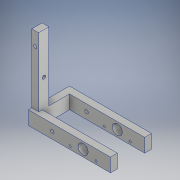
# Autodesk Inventor part: shooter
Saved by Autodesk Inventor 2019 (Build 230136000, 136)
## iProperties
Created: 2019-04-02
Part Number: shooter
Material: Aluminum 6061
Document SubType Name: Modeling
Designer: User
Density: 2.7 g/cm^3
Appearance: Aluminum - Flat
Mass: 367.89 g
Surface Area: 375.999 cm^2
Volume: 136.256 cm^3
Author: User
Autodesk Inventor part; units mm, degrees
ref_plane "YZ Plane" through (0, 0, 0) normal (1, 0, 0) x (0, 1, 0)
ref_plane "XZ Plane" through (0, 0, 0) normal (0, 1, 0) x (-1, 0, 0)
ref_plane "XY Plane" through (0, 0, 0) normal (0, 0, 1) x (1, 0, 0)
sketch "Sketch1" plane through (0, 0, 0) normal (1, 0, 0) x (0, 1, 0)
  line L0 (0, 0) -> (-152.4, 0)
  line L1 (-152.4, 0) -> (-152.4, -12.7)
  line L2 (-152.4, -12.7) -> (0, -12.7)
  line L3 (0, -12.7) -> (0, 0)
  line L4 (0, -12.7) -> (-12.7, -12.7)
  line L5 (-12.7, -12.7) -> (-12.7, -63.5)
  line L6 (-12.7, -63.5) -> (0, -63.5)
  line L7 (0, -63.5) -> (0, -12.7)
  line L8 (0, -63.5) -> (-152.4, -63.5)
  line L9 (-152.4, -63.5) -> (-152.4, -76.2)
  line L10 (-152.4, -76.2) -> (0, -76.2)
  line L11 (0, -76.2) -> (0, -63.5)
  dimension "d0" = 152.4
  dimension "d1" = 12.7
  dimension "d2" = 12.7
  dimension "d3" = 50.8
  dimension "d4" = 12.7
  dimension "d5" = 152.4
  constraints: 24 end point, 6 parallel, 3 horizontal, 3 perpendicular
  measures "d0" distance of L2.end L1.end
  measures "d1" distance of L1.end L0.end
  measures "d2" distance of L6.end L5.end
  measures "d3" distance of L5.end L4.end
  measures "d4" distance of L8.end L9.end
  measures "d5" distance of L9.end L10.end
extrude "Extrusion1" add sketch "Sketch1" along normal blind 25.4
sketch "Sketch2" plane through (0, -152.4, -76.2) normal (0, 0, -1) x (-1, 0, 0)
  line L0 (0, 152.4) -> (-25.4, 152.4) projected
  line L1 (-25.4, 0) -> (-25.4, 152.4) projected
  point P0 (-12.7, 107.95)
  dimension "d8" = 44.45
  dimension "d9" = 25.4
  dimension "d10" = 12.7
  measures "d8" distance from line of L0 point (-12.7, 107.95)
  measures "d9" distance of L0.start L0.end
  measures "d10" distance from line of L1 point (-12.7, 107.95)
hole "Hole1" at (12.7, -44.45, -76.2) direction (0, 0, 1) diameter 6.35 end through all
sketch "Sketch3" plane through (0, -152.4, -76.2) normal (0, 0, -1) x (-1, 0, 0)
  circle A0 centre (-12.7, 107.95) radius 3.175 projected
  line L0 (0, 0) -> (0, 152.4) projected
  line L1 (0, 152.4) -> (-25.4, 152.4) projected
  line L2 (-25.4, 0) -> (-25.4, 152.4) projected
  line L3 (0, 0) -> (-25.4, 0) projected
  point P0 (0, 152.4)
  point P1 (-12.7, 50.8)
  dimension "d18" = 25.4
  dimension "d19" = 12.7
  dimension "d20" = 50.8
  measures "d18" distance of L0.start L2.start
  measures "d19" distance from line of L2 point (-12.7, 50.8)
  measures "d20" distance from line of L3 point (-12.7, 50.8)
hole "Hole2" at (12.7, -101.6, -76.2) direction (0, 0, 1) diameter 18.4912 end through all
sketch "Sketch4" plane through (0, -152.4, -76.2) normal (0, 0, -1) x (-1, 0, 0)
  circle A0 centre (-12.7, 50.8) radius 9.2456 projected
  circle A1 centre (-12.7, 107.95) radius 3.175 projected
  line L0 (0, 0) -> (0, 152.4) projected
  line L1 (0, 152.4) -> (-25.4, 152.4) projected
  line L2 (-25.4, 0) -> (-25.4, 152.4) projected
  line L3 (0, 0) -> (-25.4, 0) projected
  point P0 (0, 152.4)
  point P1 (-5.6896, 26.797)
  point P2 (-5.6896, 74.803)
  dimension "d28" = 48.006
  dimension "d29" = 7.0104
  dimension "d30" = 7.0104
  dimension "d31" = 24.003
  measures "d28" distance of point (-5.69, 26.797) point (-5.69, 74.803)
  measures "d29" horizontal distance of point (-5.69, 74.803) A0.centre
  measures "d30" horizontal distance of A0.centre point (-5.69, 26.797)
  measures "d31" vertical distance of A0.centre point (-5.69, 26.797)
hole "Hole3" at (5.6896, -125.603, -76.2) at (5.6896, -77.597, -76.2) direction (0, 0, 1) diameter 3.7084 end through all
sketch "Sketch5" plane through (25.4, 0, 0) normal (1, 0, 0) x (0, 0, -1)
  line L0 (76.2, 0) -> (0, 0) projected
  line L1 (12.7, -12.7) -> (63.5, -12.7) projected
  line L2 (6.35, 0) -> (25.4, 0)
  line L3 (25.4, 0) -> (25.4, -12.7)
  line L4 (25.4, -12.7) -> (6.35, -12.7)
  line L5 (6.35, -12.7) -> (6.35, 0)
  line L6 (0, 0) -> (0, -152.4) projected
  dimension "d39" = 19.05
  dimension "d40" = 6.35
  constraints: 8 end point, 2 parallel, 2 point on line, 1 horizontal, 1 perpendicular
  measures "d39" distance of L3.end L4.end
  measures "d40" distance between parallel lines of L6 L5
extrude "Extrusion2" add sketch "Sketch5" along normal blind 127
sketch "Sketch6" plane through (0, -12.7, -63.5) normal (0, -1, 0) x (1, 0, 0)
  line L0 (0, 50.8) -> (0, 0) projected
  line L1 (0, 0) -> (25.4, 0) projected
  line L2 (25.4, 38.1) -> (25.4, 0) projected
  line L3 (25.4, 38.1) -> (152.4, 38.1) projected
  line L4 (152.4, 57.15) -> (152.4, 38.1) projected
  line L5 (25.4, 57.15) -> (152.4, 57.15) projected
  line L6 (25.4, 50.8) -> (25.4, 57.15) projected
  line L7 (0, 50.8) -> (25.4, 50.8) projected
  point P0 (0, 63.5)
  point P1 (76.2, 47.625)
  dimension "d43" = 19.05
  dimension "d44" = 9.525
  dimension "d45" = 50.8
  measures "d43" distance of L4.start L3.end
  measures "d44" distance from line of L3 point (76.2, 47.625)
  measures "d45" distance from line of L2 point (76.2, 47.625)
hole "Hole4" at (76.2, -12.7, -15.875) direction (0, 1, 0) diameter 6.35 end through all
sketch "Sketch7" plane through (25.4, -12.7, -25.4) normal (0, 0, -1) x (-1, 0, 0)
  line L0 (-47.625, 12.7) -> (-47.625, 0) projected
  line L1 (0, 12.7) -> (0, 0) projected
  line L2 (0, 12.7) -> (-127, 12.7) projected
  line L3 (-127, 0) -> (-127, 12.7) projected
  line L4 (0, 0) -> (-127, 0) projected
  line L5 (0, -139.7) -> (0, 12.7) projected
  point P0 (25.4, 12.7)
  point P1 (-101.6, 6.35)
  dimension "d53" = 12.7
  dimension "d54" = 6.35
  dimension "d55" = 101.6
  measures "d53" distance of L3.start L2.end
  measures "d54" distance from line of L2 point (-101.6, 6.35)
  measures "d55" distance from line of L5 point (-101.6, 6.35)
hole "Hole5" at (127, -6.35, -25.4) direction (0, 0, 1) diameter 6.35 end through all
equation "\"d2\" = d1"
equation "\"d4\" = d1"
equation "\"d5\" = d0"
equation "\"d10\" = 0.5 * d9"
equation "\"d19\" = 0.5 * d18"
equation "\"d30\" = d29"
equation "\"d31\" = 0.5 * d28"
equation "\"d44\" = 0.5 * d43"
equation "\"d54\" = 0.5 * d53"
body "Solid1"
